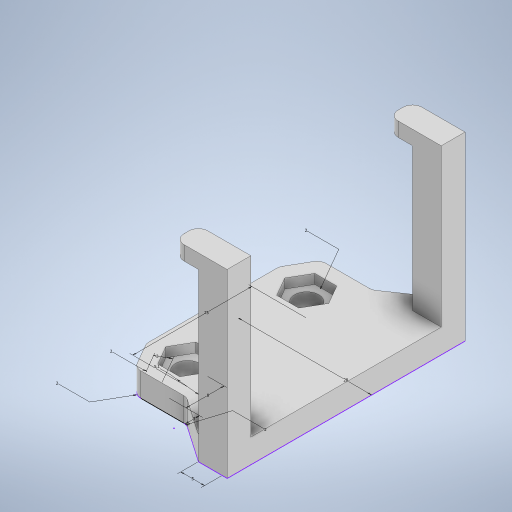
# Autodesk Inventor part: soporte_pinzas
Saved by Autodesk Inventor 2024 (Build 280153000, 153)
## iProperties
Created: 2023-06-27
Part Number: soporte_pinzas
Material: Generic
Document SubType Name: Modeling
Designer: LabTel_Admin
Density: 1 g/cm^3
Appearance: Default
Author: LabTel_Admin
Autodesk Inventor part; units mm, degrees
ref_plane "YZ Plane" through (0, 0, 0) normal (1, 0, 0) x (0, 1, 0)
ref_plane "XZ Plane" through (0, 0, 0) normal (0, 1, 0) x (-1, 0, 0)
ref_plane "XY Plane" through (0, 0, 0) normal (0, 0, 1) x (1, 0, 0)
sketch "Sketch2" plane through (0, 0, 0) normal (0, 1, 0) x (-1, 0, 0)
  line L0 (15.1065, 12.5) -> (17.4159, 16.5)
  line L1 (17.4159, 16.5) -> (22.0347, 16.5)
  line L2 (22.0347, 16.5) -> (24.3441, 12.5)
  line L3 (24.3441, 12.5) -> (22.0347, 8.5)
  line L4 (22.0347, 8.5) -> (17.4159, 8.5)
  line L5 (17.4159, 8.5) -> (15.1065, 12.5)
  circle A0 centre (19.7253, 12.5) radius 2.55
  line L6 (13.6122, 19.5) -> (22.612, 19.5)
  line L7 (24.3441, 18.5) -> (26.7031, 14.414)
  line L8 (26.9711, 13.414) -> (26.9711, 0.8204)
  line L9 (13.6122, 19.5) -> (13.6603, 19.5)
  line L10 (0, 0) -> (8.2774, 0) construction
  line L11 (15.1065, -12.5) -> (17.4159, -16.5)
  line L12 (17.4159, -16.5) -> (22.0347, -16.5)
  line L13 (22.0347, -16.5) -> (24.3441, -12.5)
  line L14 (24.3441, -12.5) -> (22.0347, -8.5)
  line L15 (22.0347, -8.5) -> (17.4159, -8.5)
  line L16 (17.4159, -8.5) -> (15.1065, -12.5)
  circle A1 centre (19.7253, -12.5) radius 2.55
  line L17 (13.6603, -19.5) -> (22.612, -19.5)
  line L18 (24.3441, -18.5) -> (26.7031, -14.414)
  line L19 (26.9711, -13.414) -> (26.9711, -0.8204)
  line L20 (13.6122, -19.5) -> (13.6603, -19.5)
  line L21 (0, 25) -> (5, 25)
  line L22 (26.9711, 0.8204) -> (26.9711, -0.8204)
  line L23 (2, 20) -> (5, 20)
  line L24 (5, 20) -> (5, 25)
  line L25 (12.4782, 19.8526) -> (5, 25)
  arc A2 (12.4782, 19.8526) -> (13.6122, 19.5) centre (13.6122, 21.5) ccw
  arc A3 (24.3441, 18.5) -> (22.612, 19.5) centre (22.612, 17.5) ccw
  arc A4 (26.9711, 13.414) -> (26.7031, 14.414) centre (24.9711, 13.414) ccw
  line L26 (0, -25) -> (5, -25)
  line L27 (2, -20) -> (5, -20)
  line L28 (5, -20) -> (5, -25)
  line L29 (12.4782, -19.8526) -> (5, -25)
  arc A5 (13.6122, -19.5) -> (12.4782, -19.8526) centre (13.6122, -21.5) ccw
  arc A6 (22.612, -19.5) -> (24.3441, -18.5) centre (22.612, -17.5) ccw
  arc A7 (26.7031, -14.414) -> (26.9711, -13.414) centre (24.9711, -13.414) ccw
  line L30 (0, -25) -> (-1.0289, -25)
  line L31 (-1.0289, -25) -> (-1.0289, 25)
  line L32 (-1.0289, 25) -> (0, 25)
  line L33 (2, 20) -> (-1.0289, 20)
  line L34 (2, -20) -> (-1.0289, -20)
  point P0 (3, 23.2679)
  point P1 (19.7253, 8.5)
  point P2 (19.7253, 16.5)
  point P3 (23.7667, 19.5)
  point P4 (26.9711, 13.9499)
  point P5 (23.1894, 14.5)
  point P6 (12.9904, 19.5)
  point P7 (19.7253, -8.5)
  point P8 (19.7253, -16.5)
  point P9 (23.7667, -19.5)
  point P10 (26.9711, -13.9499)
  point P11 (23.1894, -14.5)
  point P12 (12.9904, -19.5)
  point P13 (25.239, 0.1796)
  point P14 (25.239, -0.1796)
  dimension "d18" = 8
  dimension "d19" = 5.1
  dimension "d21" = 3
  dimension "d22" = 3
  dimension "d27" = 25
  dimension "d33" = 5
  dimension "d34" = 2
  dimension "d35" = 2
  dimension "d36" = 2
  dimension "d37" = 2
  dimension "d48" = 28
  constraints: 70 end point, 23 symmetric about line, 13 point on line, 12 point on circle, 10 tangent, 8 centre point, 6 horizontal, 5 perpendicular, 3 midpoint, 2 coincident, 2 vertical, 1 equal radius, 1 parallel, 15 other
  measures "d18" distance of point (19.725, 8.5) point (19.725, 16.5)
  measures "d19" diameter of A0
  measures "d21" distance between parallel lines of L6 L1
  measures "d22" distance from line of L7 point (23.189, 14.5)
  measures "d27" distance of point (19.725, -12.5) point (19.725, 12.5)
  measures "d33" distance of L21.start L21.end
  measures "d34" radius of A2
  measures "d35" radius of A3
  measures "d36" radius of A4
  measures "d37" radius of A6
  measures "d48" distance between parallel lines of L31 L19
extrude "Extrusion2" add sketch "Sketch2" along normal blind 35 contours L24 L23 L33 L31 L32 L21
extrude "Extrusion4" add sketch "Sketch2" along normal blind 3 contours L0 L1 L2 L3 L4 L5 | L16 L15 L14 L13 L12 L11
extrude "Extrusion6" add sketch "Sketch2" along normal blind 5 contours L6 A3 L7 A4 L8 L22 L19 A7 L18 A6 L17 L20 A5 L29 L28 L27 L34 L31 L33 L23 L24 L25 A2
extrude "Extrusion7" add sketch "Sketch2" along normal blind 35 contours L34 L27 L28 L26 L30 L31
sketch "Sketch4" plane through (0, 35, 0) normal (0, 1, 0) x (1, 0, 0)
  line L0 (-5, -25) -> (1.0289, -25) projected
  line L1 (0, -25) -> (-8, -25)
  line L2 (-10, -23) -> (-10, -22)
  line L3 (-8, -20) -> (0, -20)
  line L4 (0, 0) -> (-6.9228, 0) construction
  line L5 (0, 25) -> (-8, 25)
  line L6 (-10, 23) -> (-10, 22)
  line L7 (-8, 20) -> (0, 20)
  arc A0 (-10, -23) -> (-8, -25) centre (-8, -23) ccw
  arc A1 (-8, -20) -> (-10, -22) centre (-8, -22) ccw
  arc A2 (-10, 22) -> (-8, 20) centre (-8, 22) ccw
  arc A3 (-8, 25) -> (-10, 23) centre (-8, 23) ccw
  line L8 (1.0289, -20) -> (-5, -20) projected
  line L9 (0, -20) -> (1.0289, -20)
  line L10 (1.0289, -20) -> (1.0289, -25)
  line L11 (0, -25) -> (1.0289, -25)
  line L12 (-5, 20) -> (1.0289, 20) projected
  line L13 (0, 20) -> (1.0289, 20)
  line L14 (1.0289, 20) -> (1.0289, 25)
  line L15 (1.0289, 25) -> (0, 25)
  point P0 (-10, -20)
  point P1 (-10, -25)
  point P2 (-10, 20)
  point P3 (-10, 25)
  dimension "d42" = 10
  dimension "d43" = 5
  dimension "d44" = 2
  constraints: 26 end point, 8 point on circle, 8 point on line, 8 tangent, 5 perpendicular, 4 centre point, 4 symmetric about line, 3 equal radius, 2 horizontal, 1 parallel
  measures "d42" distance of point (-10, -20) L3.end
  measures "d43" distance of point (-10, -25) point (-10, -20)
  measures "d44" radius of A0
extrude "Extrusion8" add sketch "Sketch4" along normal blind 3
body "Solid1"
